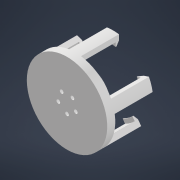
# Autodesk Inventor part: tire disk
Saved by Autodesk Inventor 2022 (Build 260153000, 153)
## iProperties
Created: 2023-02-07
Part Number: tire disk
Material: Типовые
Document SubType Name: Modeling
Designer: akapu
Density: 1 g/cm^3
Appearance: По умолчанию
Author: akapu
Autodesk Inventor part; units mm, degrees
ref_plane "YZ Plane" through (0, 0, 0) normal (1, 0, 0) x (0, 1, 0)
ref_plane "XZ Plane" through (0, 0, 0) normal (0, 1, 0) x (-1, 0, 0)
ref_plane "XY Plane" through (0, 0, 0) normal (0, 0, 1) x (1, 0, 0)
sketch "Эскиз1" plane through (0, 0, 0) normal (0, 0, 1) x (1, 0, 0)
  circle A0 centre (0, 0) radius 21.25 projected
  circle A1 centre (0, 0) radius 30 projected
  circle A2 centre (0, 0) radius 21.25
  circle A3 centre (0, 0) radius 30
  circle A4 centre (0, 0) radius 35
  line L0 (0, 0) -> (6.0777, 34.4683)
  line L1 (0, 0) -> (35, 0) construction
  line L2 (0, 0) -> (-6.0777, 34.4683)
  line L3 (0, 0) -> (35, 0) construction
  line L4 (-5.2094, 29.5442) -> (-5.2094, 34.6101)
  line L5 (5.2094, 29.5442) -> (5.2094, 34.6101)
  line L6 (-26.4884, 14.0841) -> (-31.3064, 15.6496)
  line L7 (-29.708, 4.1752) -> (-34.526, 5.7406)
  line L8 (-21.5802, -20.8398) -> (-24.5579, -24.9382)
  line L9 (-13.1511, -26.9638) -> (-16.1288, -31.0622)
  line L10 (13.1511, -26.9638) -> (16.1288, -31.0622)
  line L11 (21.5802, -20.8398) -> (24.5579, -24.9382)
  line L12 (29.708, 4.1752) -> (34.526, 5.7406)
  line L13 (26.4884, 14.0841) -> (31.3064, 15.6496)
  circle A5 centre (0, 0) radius 30.4
  point P0 (0, 0)
  point P1 (5.2094, 29.5442)
  point P2 (-5.2094, 29.5442)
  point P3 (-5.2094, 29.9503)
  point P4 (5.2094, 29.9503)
  point P5 (26.8746, 14.2096)
  point P6 (30.0943, 4.3007)
  point P7 (-30.0943, 4.3007)
  point P8 (-26.8746, 14.2096)
  point P9 (-13.3898, -27.2924)
  point P10 (-21.8189, -21.1683)
  point P11 (21.8189, -21.1683)
  point P12 (13.3898, -27.2924)
  dimension "d0" = 70
  dimension "d1" = 80
  dimension "d2" = 100
  dimension "d5" = 360
  dimension "d19" = 0.4
  constraints: 28 end point, 6 point on circle, 4 centre point, 3 coincident, 2 concentric, 2 equal length, 2 horizontal, 2 point on line, 1 vertical, 31 other
  measures "d0" diameter of A4
  measures "d1" angle of L1 L0
  measures "d2" angle of L3 L2
  measures "d19" radial gap between concentric circles of A1 A5
extrude "Выдавливание1" add sketch "Эскиз1" against normal blind 33 contours A0 L2 L0 | L0 L2 A0 | A5 L4 A4 L5 | L13 A4 L12 A5 | A5 L7 A4 L6 | A5 L9 A4 L8 | L11 A4 L10 A5
sketch "Эскиз2" plane through (0, 0, 0) normal (1, 0, 0) x (0, 1, 0)
  line L0 (30, -23) -> (30, 0) projected
  line L1 (-30, -19.93) -> (30, -19.93) projected
  line L2 (0, 0) -> (0, -33)
  line L3 (-21.25, -33) -> (21.25, -33) projected
  line L4 (22.45, -18.73) -> (21.25, -17.53)
  line L5 (22.45, -19.93) -> (22.45, -18.73)
  line L6 (21.25, 0) -> (21.25, -33) projected
  line L7 (-30, -19.93) -> (30, -19.93) projected
  line L8 (21.25, -2.4) -> (22.45, -1.2)
  line L9 (22.45, -1.2) -> (22.45, 0)
  line L10 (30, 0) -> (-30, 0) projected
  line L11 (30.4, -33) -> (30.4, 0) projected
  line L12 (30.4, -33) -> (30.4, 0) projected
  line L13 (30.4, -33) -> (30.4, 0) projected
  line L14 (-30, -29.93) -> (30, -29.93) projected
  line L15 (20.7199, -30.23) -> (27.0363, -30.23) projected
  line L16 (30.4, -33) -> (30.4, 0) projected
  line L17 (30.4, -33) -> (30.4, -30.1)
  line L18 (30.4, -33) -> (30.4, 0) projected
  line L19 (30.4, -30.1) -> (26.4, -30.1)
  line L20 (26.4, -30.1) -> (26.4, -30.5)
  line L21 (26.4, -30.1) -> (26.8, -30.1) construction
  line L22 (26.4, -30.5) -> (30.4, -33)
  point P0 (21.25, -19.93)
  dimension "d25" = 2.9
  dimension "d26" = 4
  dimension "d27" = 0.4
  dimension "d28" = 90
  constraints: 20 end point, 3 vertical, 2 horizontal, 1 midpoint, 1 perpendicular, 11 other
  measures "d25" distance of L16.start L17.end
  measures "d26" distance of L17.end L19.end
  measures "d27" distance of L19.end L20.end
  measures "d28" angle of L20 L21
revolve "Вращение1" add sketch "Эскиз2" angle 360 about axis through (0, 0, 0) along (0, 0, -1) contours L20 L19 L11 L22 | L1 L6 L4 L5 | L9 L8 L6 L10
sketch "Эскиз3" plane through (0, 0, -33) normal (0, 0, -1) x (-1, 0, 0)
  arc A0 (5.2094, 34.6101) -> (-5.2094, 34.6101) centre (0, 0) ccw projected
  line L0 (-5.2094, 34.6101) -> (-5.2094, 26.4927)
  line L1 (5.2094, 34.6101) -> (5.2094, 26.4927)
  circle A1 centre (0, 0) radius 35
  line L2 (-31.3064, 15.6496) -> (-23.5862, 13.1412)
  line L3 (-34.526, 5.7406) -> (-26.8058, 3.2322)
  line L4 (-24.5579, -24.9382) -> (-19.7865, -18.371)
  line L5 (-16.1288, -31.0622) -> (-11.3575, -24.4951)
  line L6 (16.1288, -31.0622) -> (11.3575, -24.4951)
  line L7 (24.5579, -24.9382) -> (19.7865, -18.371)
  line L8 (34.526, 5.7406) -> (26.8058, 3.2322)
  line L9 (31.3064, 15.6496) -> (23.5862, 13.1412)
  circle A2 centre (0, 0) radius 27
  point P0 (0, 0)
  point P1 (5.2094, 34.6101)
  point P2 (5.2094, 34.6101)
  dimension "d13" = 360
  constraints: 20 end point, 2 coincident, 2 vertical, 37 other
extrude "Выдавливание2" cut sketch "Эскиз3" against normal blind 23 contours A1 L9 A2 L1 | L0 A2 L2 A1 | A2 | A1 L7 A2 L8 | L3 A2 L4 A1 | L5 A2 L6 A1
sketch "Эскиз4" plane through (0, 0, 0) normal (0, 0, 1) x (1, 0, 0)
  arc A0 (5.2094, 34.6101) -> (-5.2094, 34.6101) centre (0, 0) ccw projected
  circle A1 centre (0, 0) radius 35
  point P0 (0, 0)
  point P1 (5.2094, 34.6101)
  constraints: 1 coincident, 3 other
extrude "Выдавливание3" add sketch "Эскиз4" along normal blind 7
sketch "Эскиз5" plane through (0, 0, 0) normal (1, 0, 0) x (0, 1, 0)
  line L0 (-21.25, -10) -> (21.25, -10) projected
  line L1 (21.25, -10) -> (-21.25, -10) projected
  line L2 (21.25, -10) -> (18.75, -10)
  line L3 (18.75, -10) -> (16.6287, -12.1213)
  line L4 (16.6287, -12.1213) -> (0, -12.1213)
  line L5 (14.2096, 0) -> (14.2096, -30.1) projected
  line L6 (0, -12.1213) -> (0, -10)
  point P0 (0, 0)
  dimension "d29" = 2.5
  dimension "d30" = 3
  dimension "d31" = 135
  constraints: 8 end point, 1 midpoint, 1 perpendicular, 1 point on line
  measures "d29" distance of L0.end L2.end
  measures "d30" distance of L2.end L3.end
  measures "d31" angle of L3 L2
revolve "Вращение2" add sketch "Эскиз5" angle 360 about axis through (0, 0, -12.1213) along (0, 0, 1)
sketch "Эскиз6" plane through (0, 0, 0) normal (1, 0, 0) x (0, 1, 0)
  line L0 (25.52, -29.93) -> (25.52, 0)
  line L1 (25.52, 0) -> (25.52, 2)
  line L2 (30.4, -30.1) -> (30.4, 0) projected
  line L3 (29.9503, 0) -> (29.9503, -30.1) projected
  line L4 (25.52, 2) -> (29.9503, 0)
  line L5 (30.1003, -30.1) -> (30.1003, 0.0969)
  line L6 (30.1003, 0.0969) -> (25.37, 2.2323)
  line L7 (25.37, 2.2323) -> (25.37, 0)
  line L8 (25.37, 0) -> (25.37, -29.93)
  line L9 (35, 7) -> (-35, 7) projected
  line L10 (0, 7) -> (0, 0)
  line L11 (25.37, 0) -> (30.3149, 0)
  line L12 (34.6101, 0) -> (15.6496, 0) projected
  point P0 (30.1003, 0)
  dimension "d33" = 0.15
  constraints: 18 end point, 3 vertical, 2 point on line, 1 midpoint, 5 other
  measures "d33" distance between parallel lines of L4 L6
revolve "Вращение3" cut sketch "Эскиз6" angle 360 about axis through (0, 0, 7) along (0, 0, -1)
sketch "Эскиз7" plane through (0, 0, -12.1213) normal (0, 0, -1) x (-1, 0, 0)
  line L0 (15.0382, 14.3621) -> (21.6953, 20.7199) projected
  arc A0 (21.6953, 20.7199) -> (13.0016, 27.0363) centre (0, 0) ccw projected
  line L1 (13.0016, 27.0363) -> (9.0121, 18.7403) projected
  arc A1 (-9.0121, 18.7403) -> (9.0121, 18.7403) centre (0, 23.0741) ccw projected
  line L2 (-9.0121, 18.7403) -> (-13.0016, 27.0363) projected
  arc A2 (-13.0016, 27.0363) -> (-21.6953, 20.7199) centre (0, 0) ccw projected
  line L3 (-21.6953, 20.7199) -> (-15.0382, 14.3621) projected
  arc A3 (-20.608, -2.7799) -> (-15.0382, 14.3621) centre (-21.9448, 7.1303) ccw projected
  line L4 (-20.608, -2.7799) -> (-29.7307, -4.0106) projected
  arc A4 (-29.7307, -4.0106) -> (-26.41, -14.2307) centre (0, 0) ccw projected
  line L5 (-26.41, -14.2307) -> (-18.3062, -9.864) projected
  arc A5 (-3.7243, -20.4584) -> (-18.3062, -9.864) centre (-13.5626, -18.6674) ccw projected
  line L6 (-3.7243, -20.4584) -> (-5.373, -29.5149) projected
  arc A6 (-5.373, -29.5149) -> (5.373, -29.5149) centre (0, 0) ccw projected
  line L7 (5.373, -29.5149) -> (3.7243, -20.4584) projected
  arc A7 (18.3062, -9.864) -> (3.7243, -20.4584) centre (13.5626, -18.6674) ccw projected
  line L8 (18.3062, -9.864) -> (26.41, -14.2307) projected
  arc A8 (26.41, -14.2307) -> (29.7307, -4.0106) centre (0, 0) ccw projected
  line L9 (29.7307, -4.0106) -> (20.608, -2.7799) projected
  arc A9 (15.0382, 14.3621) -> (20.608, -2.7799) centre (21.9448, 7.1303) ccw projected
  circle A10 centre (-4.7023, 6.4721) radius 1.6 projected
  circle A11 centre (0, 0) radius 1.6 projected
  circle A12 centre (0, -8) radius 1.6 projected
  circle A13 centre (4.7023, 6.4721) radius 1.6 projected
  circle A14 centre (7.6085, -2.4721) radius 1.6 projected
  circle A15 centre (-7.6085, -2.4721) radius 1.6 projected
  line L10 (15.0382, 14.3621) -> (21.6953, 20.7199) projected
  arc A16 (21.6953, 20.7199) -> (13.0016, 27.0363) centre (0, 0) ccw projected
  line L11 (13.0016, 27.0363) -> (9.0121, 18.7403) projected
  arc A17 (-9.0121, 18.7403) -> (9.0121, 18.7403) centre (0, 23.0741) ccw projected
  line L12 (-9.0121, 18.7403) -> (-13.0016, 27.0363) projected
  arc A18 (-13.0016, 27.0363) -> (-21.6953, 20.7199) centre (0, 0) ccw projected
  line L13 (-21.6953, 20.7199) -> (-15.0382, 14.3621) projected
  arc A19 (-20.608, -2.7799) -> (-15.0382, 14.3621) centre (-21.9448, 7.1303) ccw projected
  line L14 (-20.608, -2.7799) -> (-29.7307, -4.0106) projected
  arc A20 (-29.7307, -4.0106) -> (-26.41, -14.2307) centre (0, 0) ccw projected
  line L15 (-26.41, -14.2307) -> (-18.3062, -9.864) projected
  arc A21 (-3.7243, -20.4584) -> (-18.3062, -9.864) centre (-13.5626, -18.6674) ccw projected
  line L16 (-3.7243, -20.4584) -> (-5.373, -29.5149) projected
  arc A22 (-5.373, -29.5149) -> (5.373, -29.5149) centre (0, 0) ccw projected
  line L17 (5.373, -29.5149) -> (3.7243, -20.4584) projected
  arc A23 (18.3062, -9.864) -> (3.7243, -20.4584) centre (13.5626, -18.6674) ccw projected
  line L18 (18.3062, -9.864) -> (26.41, -14.2307) projected
  arc A24 (26.41, -14.2307) -> (29.7307, -4.0106) centre (0, 0) ccw projected
  line L19 (29.7307, -4.0106) -> (20.608, -2.7799) projected
  arc A25 (15.0382, 14.3621) -> (20.608, -2.7799) centre (21.9448, 7.1303) ccw projected
  point P0 (0, 0)
extrude "Выдавливание4" cut sketch "Эскиз7" against normal up to surface (19.1213 mm away) contours A10 | A11 | A12 | A13 | A14 | A15
sketch "Эскиз8" plane through (0, 0, 7) normal (0, 0, 1) x (1, 0, 0)
  circle A0 centre (0, 0) radius 1.6 projected
  line L0 (0, 0) -> (0, 2.7)
  circle A1 centre (0, -8) radius 1.6 projected
  line L1 (0, -8) -> (0, -5.3)
  line L2 (1.5588, -5.3) -> (3.1177, -8)
  line L3 (3.1177, -8) -> (1.5588, -10.7)
  line L4 (1.5588, -10.7) -> (-1.5588, -10.7)
  line L5 (-1.5588, -10.7) -> (-3.1177, -8)
  line L6 (-3.1177, -8) -> (-1.5588, -5.3)
  line L7 (-1.5588, -5.3) -> (1.5588, -5.3)
  line L8 (1.5588, 2.7) -> (3.1177, 0)
  line L9 (3.1177, 0) -> (1.5588, -2.7)
  line L10 (1.5588, -2.7) -> (-1.5588, -2.7)
  line L11 (-1.5588, -2.7) -> (-3.1177, 0)
  line L12 (-3.1177, 0) -> (-1.5588, 2.7)
  line L13 (-1.5588, 2.7) -> (1.5588, 2.7)
  line L14 (4.5589, -3.1203) -> (5.5223, -0.1552)
  line L15 (7.6085, -2.4721) -> (5.0406, -1.6378)
  line L16 (6.645, -5.4372) -> (4.5589, -3.1203)
  line L17 (9.6946, -4.789) -> (6.645, -5.4372)
  line L18 (10.658, -1.8239) -> (9.6946, -4.789)
  line L19 (8.5719, 0.493) -> (10.658, -1.8239)
  line L20 (5.5223, -0.1552) -> (8.5719, 0.493)
  line L21 (4.3764, 3.3715) -> (1.8541, 5.2041)
  line L22 (4.7023, 6.4721) -> (3.1153, 4.2878)
  line L23 (7.2245, 4.6396) -> (4.3764, 3.3715)
  line L24 (7.5504, 7.7402) -> (7.2245, 4.6396)
  line L25 (5.0282, 9.5727) -> (7.5504, 7.7402)
  line L26 (2.18, 8.3047) -> (5.0282, 9.5727)
  line L27 (1.8541, 5.2041) -> (2.18, 8.3047)
  line L28 (-1.8541, 5.2041) -> (-4.3764, 3.3715)
  line L29 (-4.7023, 6.4721) -> (-3.1153, 4.2878)
  line L30 (-2.18, 8.3047) -> (-1.8541, 5.2041)
  line L31 (-5.0282, 9.5727) -> (-2.18, 8.3047)
  line L32 (-7.5504, 7.7402) -> (-5.0282, 9.5727)
  line L33 (-7.2245, 4.6396) -> (-7.5504, 7.7402)
  line L34 (-4.3764, 3.3715) -> (-7.2245, 4.6396)
  line L35 (-5.5223, -0.1552) -> (-4.5589, -3.1203)
  line L36 (-7.6085, -2.4721) -> (-5.0406, -1.6378)
  line L37 (-8.5719, 0.493) -> (-5.5223, -0.1552)
  line L38 (-10.658, -1.8239) -> (-8.5719, 0.493)
  line L39 (-9.6946, -4.789) -> (-10.658, -1.8239)
  line L40 (-6.645, -5.4372) -> (-9.6946, -4.789)
  line L41 (-4.5589, -3.1203) -> (-6.645, -5.4372)
  point P0 (0, 0)
  dimension "d40" = 2.7
  dimension "d41" = 2.7
  dimension "d44" = 360
  constraints: 84 end point, 6 coincident, 2 midpoint, 2 vertical, 107 other
  measures "d40" distance of L0.start L0.end
  measures "d41" distance of L1.start L1.end
extrude "Выдавливание5" cut sketch "Эскиз8" against normal blind 4
